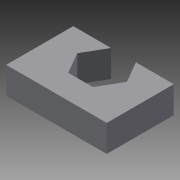
# Autodesk Inventor part: piulita telescop
Saved by Autodesk Inventor 2015 SP1 (Build 190203100, 203)
## iProperties
Created: 2015-05-10
Part Number: piulita telescop
Material: Generic
Document SubType Name: Modeling
Designer: ubik
Density: 1 g/cm^3
Appearance: Default
Author: ubik
Autodesk Inventor part; units mm, degrees
ref_plane "YZ Plane" through (0, 0, 0) normal (1, 0, 0) x (0, 1, 0)
ref_plane "XZ Plane" through (0, 0, 0) normal (0, 1, 0) x (-1, 0, 0)
ref_plane "XY Plane" through (0, 0, 0) normal (0, 0, 1) x (1, 0, 0)
sketch "Sketch1" plane through (0, 0, 0) normal (0, 0, 1) x (1, 0, 0)
  line L0 (0, 0) -> (30, 0)
  line L1 (30, 0) -> (30, 20)
  line L2 (30, 20) -> (0, 20)
  line L3 (0, 20) -> (0, 0)
  line L4 (11.305, 7.2) -> (7.6099, 13.6)
  line L5 (7.6099, 13.6) -> (11.305, 20)
  line L6 (11.305, 20) -> (18.695, 20)
  line L7 (18.695, 20) -> (22.3901, 13.6)
  line L8 (22.3901, 13.6) -> (18.695, 7.2)
  line L9 (18.695, 7.2) -> (11.305, 7.2)
  point P0 (15, 13.6)
  dimension "d0" = 30
  dimension "d1" = 20
  dimension "d2" = 12.8
  dimension "d3" = 0
  dimension "d4" = 15
  constraints: 20 end point, 2 parallel, 1 horizontal, 1 perpendicular, 13 other
  measures "d0" distance of L2.end L1.end
  measures "d1" distance of L1.end L0.end
  measures "d2" distance between parallel lines of L6 L9
  measures "d3" distance between parallel lines of L2 L6
  measures "d4" distance from line of point (15, 13.6) L3
extrude "Extrusion1" add sketch "Sketch1" along normal blind 8 contours L3 L2 L5 L4 L9 L8 L7 L1 L0
body "Solid1"
